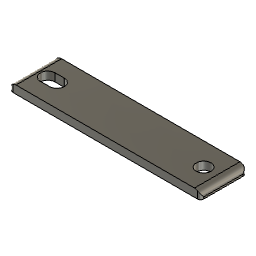
foldable phone springs (Autodesk Fusion 360 design; units mm, degrees)
Autodesk Fusion 360 part; units mm, degrees
sketch "Sketch1" plane through (0, 0, 0) normal (0, 0, 1) x (1, 0, 0)
  line L0 (-31, 7.4) -> (31, 7.4)
  line L1 (31, 7.4) -> (31, -7.4)
  line L2 (31, -7.4) -> (-31, -7.4)
  line L3 (-31, -7.4) -> (-31, 7.4)
  line L4 (-31, 0) -> (31, 0) construction
  circle A0 centre (24.6, 0) radius 2.4
  line L5 (0, 7.4) -> (0, -7.4) construction
  circle A1 centre (-24.6, 0) radius 2.4 construction
  line L6 (-26.1, -2.4) -> (-23.1, -2.4)
  arc A2 (-23.1, -2.4) -> (-23.1, 2.4) centre (-23.1, 0) ccw
  line L7 (-23.1, 2.4) -> (-26.1, 2.4)
  arc A3 (-26.1, 2.4) -> (-26.1, -2.4) centre (-26.1, 0) ccw
  line L8 (-26.1, 0) -> (-23.1, 0) construction
  point P0 (-24.6, 0)
  dimension "d1" = 62
  dimension "d2" = 14.8
  dimension "d3" = 4.8
  dimension "d4" = 49.2
  dimension "d5" = 3
  constraint horizontal L0
  constraint vertical L1
  constraint horizontal L2
  constraint vertical L3
  constraint midpoint L3 L4.start
  constraint midpoint L1 L4.end
  constraint coincident origin L4
  constraint coincident L4 A0.centre
  constraint midpoint L0 L5.start
  constraint midpoint L2 L5.end
  constraint symmetric A0 L5 A1
  constraint coincident origin L5
  constraint tangent L6 A2
  constraint tangent A2 L7
  constraint parallel L6 L7
  constraint tangent L7 A3
  constraint tangent L6 A3
  constraint coincident L4 A2.centre
  constraint parallel L4 L8
  constraint coincident P0 A1.centre
  constraint midpoint L8 P0
  constraint tangent A1 L7
  measures "d1" distance of L0.start L0.end
  measures "d2" distance of L0.start L2.end
  measures "d3" diameter of A0
  measures "d4" distance of A0.centre P0
  measures "d5" distance of A3.centre A2.centre
extrude "Extrude1" add sketch "Sketch1" along normal blind 2.6
fillet "Fillet2" radius 1 4 edges at (31, -7.4, 1.3) (31, 7.4, 1.3) (-31, 7.4, 1.3) (-31, -7.4, 1.3)
fillet "Fillet2" radius 2 2 edges at (31, 0, 2.6) (-31, 0, 2.6)
